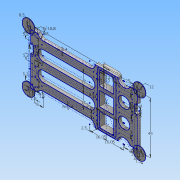
# Autodesk Inventor part: Core_top-im
Saved by Autodesk Inventor 2016 (Build 200138000, 138)
## iProperties
Created: 2015-08-27
Part Number: Core_top-im
Material: Generic
Document SubType Name: Modeling
Designer: Openlab
Density: 1 g/cm^3
Appearance: Default
Mass: 6.14664 g
Surface Area: 82.7104 cm^2
Volume: 6.14664 cm^3
Author: Openlab
Autodesk Inventor part; units mm, degrees
ref_plane "YZ Plane" through (0, 0, 0) normal (1, 0, 0) x (0, 1, 0)
ref_plane "XZ Plane" through (0, 0, 0) normal (0, 1, 0) x (-1, 0, 0)
ref_plane "XY Plane" through (0, 0, 0) normal (0, 0, 1) x (1, 0, 0)
sketch "Sketch1" plane through (0, 0, 0) normal (0, 1, 0) x (-1, 0, 0)
  line L0 (6.75, 23.75) -> (-6.75, 23.75)
  line L1 (-6.75, 23.75) -> (-6.75, 10.25)
  line L2 (-6.75, 10.25) -> (6.75, 10.25)
  line L3 (6.75, 10.25) -> (6.75, 23.75)
  line L4 (56.9183, 17) -> (21.35, 17) construction
  line L5 (69.8, -24.5) -> (69.8, -20.1) construction
  line L6 (-26.8, 24.5) -> (-26.8, -24.5) construction
  line L7 (9.25, 15.5) -> (6.75, 15.5) construction
  line L8 (6.75, 18.5) -> (9.25, 18.5) construction
  line L9 (-6.75, 15.5) -> (-9.25, 15.5) construction
  line L10 (-9.25, 18.5) -> (-6.75, 18.5) construction
  line L11 (-12.05, 18.5) -> (-24.5, 18.5) construction
  line L12 (-12.05, 15.5) -> (-24.5, 15.5) construction
  line L13 (-31, 8.5) -> (74, 8.5) construction
  line L14 (67.5, 20.5) -> (66, 20.5) construction
  line L15 (66, 13.5) -> (67.5, 13.5) construction
  line L16 (-31, 26) -> (-31, -26) construction
  line L17 (21.35, -8.5) -> (74, -8.5) construction
  line L18 (0, 20.0147) -> (0, -26) construction
  line L19 (56.8064, 0) -> (21.35, 0) construction
  line L20 (-6.75, 6.75) -> (-6.75, -6.75)
  line L21 (6.75, 6.75) -> (-6.75, 6.75)
  line L22 (6.75, -6.75) -> (6.75, 6.75)
  line L23 (-6.75, -6.75) -> (6.75, -6.75)
  line L24 (6.75, 1.5) -> (9.25, 1.5) construction
  line L25 (9.25, -1.5) -> (6.75, -1.5) construction
  line L26 (67.5, 3.5) -> (66, 3.5) construction
  line L27 (66, -3.5) -> (67.5, -3.5) construction
  line L28 (-6.75, -10.25) -> (-6.75, -23.75)
  line L29 (6.75, -10.25) -> (-6.75, -10.25)
  line L30 (6.75, -23.75) -> (6.75, -10.25)
  line L31 (-6.75, -23.75) -> (6.75, -23.75)
  line L32 (56.3008, -17) -> (21.35, -17) construction
  line L33 (67.5, -13.5) -> (66, -13.5) construction
  line L34 (66, -20.5) -> (67.5, -20.5) construction
  line L35 (9.25, -18.5) -> (6.75, -18.5) construction
  line L36 (6.75, -15.5) -> (9.25, -15.5) construction
  line L37 (74, 5) -> (72.5, 5) construction
  line L38 (69.8, 12) -> (72.5, 12) construction
  line L39 (-9.25, -15.5) -> (-6.75, -15.5) construction
  line L40 (-6.75, -18.5) -> (-9.25, -18.5) construction
  line L41 (-12.05, -18.5) -> (-24.5, -18.5) construction
  line L42 (-9.25, 1.5) -> (-6.75, 1.5) construction
  line L43 (-6.75, -1.5) -> (-9.25, -1.5) construction
  line L44 (-12.05, -1.5) -> (-24.5, -1.5) construction
  line L45 (-29.5, 5) -> (-31, 5) construction
  line L46 (-31, 12) -> (-29.5, 12) construction
  line L47 (67.5, 5.5) -> (66, 5.5) construction
  line L48 (66, 5.5) -> (66, 11.5) construction
  line L49 (66, 11.5) -> (67.5, 11.5) construction
  line L50 (-24.5, 5.5) -> (-23.5, 5.5) construction
  line L51 (-23.5, 5.5) -> (-23.5, 11.5) construction
  line L52 (-23.5, 11.5) -> (-24.5, 11.5) construction
  line L53 (-25, 24.5) -> (-25, 19) construction
  line L54 (-25, 5) -> (-25, 2) construction
  arc A0 (16.05, 13.5) -> (16.05, 3.5) centre (16.05, 8.5) ccw
  arc A1 (60, 3.5) -> (60, 13.5) centre (60, 8.5) ccw
  arc A2 (16.05, -3.5) -> (16.05, -13.5) centre (16.05, -8.5) ccw
  arc A3 (60, -13.5) -> (60, -3.5) centre (60, -8.5) ccw
  line L55 (16.05, 13.5) -> (60, 13.5)
  line L56 (16.05, 3.5) -> (60, 3.5)
  line L57 (16.05, -3.5) -> (60, -3.5)
  line L58 (16.05, -13.5) -> (60, -13.5)
  arc A4 (-16.05, -13.5) -> (-16.05, -3.5) centre (-16.05, -8.5) ccw
  line L59 (72.5, -24.5) -> (72.5, -19.6) construction
  line L60 (-29.5, 24.5) -> (-29.5, 12) construction
  arc A5 (-17, -3.5) -> (-17, -13.5) centre (-17, -8.5) ccw
  arc A6 (-17, 13.5) -> (-17, 3.5) centre (-17, 8.5) ccw
  line L61 (-16.05, -13.5) -> (-17, -13.5)
  line L62 (-17, -3.5) -> (-16.05, -3.5)
  line L63 (-17, 3.5) -> (-16.05, 3.5)
  line L64 (-16.05, 13.5) -> (-17, 13.5)
  arc A7 (-16.05, 3.5) -> (-16.05, 13.5) centre (-16.05, 8.5) ccw
  line L65 (58.8763, -15.5) -> (12.05, -15.5) construction
  line L66 (58.8763, -18.5) -> (12.05, -18.5) construction
  line L67 (58.8763, -1.5) -> (12.05, -1.5) construction
  line L68 (58.8763, 1.5) -> (12.05, 1.5) construction
  line L69 (58.8763, 15.5) -> (12.05, 15.5) construction
  line L70 (58.8763, 18.5) -> (12.05, 18.5) construction
  arc A8 (61, -14.4) -> (58.8763, -15.5) centre (61, -17) ccw construction
  arc A9 (58.8763, -18.5) -> (61, -19.6) centre (61, -17) ccw construction
  arc A10 (61, 2.6) -> (58.8763, 1.5) centre (61, 0) ccw construction
  arc A11 (58.8763, -1.5) -> (61, -2.6) centre (61, 0) ccw construction
  arc A12 (61, 19.6) -> (58.8763, 18.5) centre (61, 17) ccw construction
  arc A13 (58.8763, 15.5) -> (61, 14.4) centre (61, 17) ccw construction
  arc A14 (63.5, -26) -> (60, -22.5) centre (60, -26) ccw construction
  arc A15 (16.05, -22.5) -> (12.55, -26) centre (16.05, -26) ccw construction
  arc A16 (64.7697, -24.5) -> (60, -21) centre (60, -26) ccw construction
  line L71 (60, -21) -> (16.05, -21) construction
  line L72 (63.5, -26) -> (74, -26) construction
  line L73 (60, -22.5) -> (16.05, -22.5) construction
  arc A17 (16.05, -21) -> (11.2803, -24.5) centre (16.05, -26) ccw construction
  arc A18 (11.2803, 24.5) -> (16.05, 21) centre (16.05, 26) ccw construction
  arc A19 (12.55, 26) -> (16.05, 22.5) centre (16.05, 26) ccw construction
  line L74 (60, 22.5) -> (16.05, 22.5) construction
  line L75 (60, 21) -> (16.05, 21) construction
  line L76 (64.7697, 24.5) -> (69.8, 24.5) construction
  line L77 (74, 26) -> (63.5, 26) construction
  arc A20 (60, 22.5) -> (63.5, 26) centre (60, 26) ccw construction
  arc A21 (60, 21) -> (64.7697, 24.5) centre (60, 26) ccw construction
  arc A22 (-12.55, -26) -> (-16.05, -22.5) centre (-16.05, -26) ccw construction
  arc A23 (-17, -22.5) -> (-20.5, -26) centre (-17, -26) ccw construction
  line L78 (-16.05, -21) -> (-17, -21) construction
  line L79 (-16.05, -22.5) -> (-17, -22.5) construction
  arc A24 (-17, -21) -> (-21.7697, -24.5) centre (-17, -26) ccw construction
  arc A25 (-11.2803, -24.5) -> (-16.05, -21) centre (-16.05, -26) ccw construction
  line L80 (11.2803, -24.5) -> (-11.2803, -24.5) construction
  line L81 (-21.7697, -24.5) -> (-29.5, -24.5) construction
  line L82 (-31, -26) -> (-20.5, -26) construction
  line L83 (-12.55, -26) -> (12.55, -26) construction
  line L84 (-16.05, 21) -> (-17, 21) construction
  line L85 (-16.05, 22.5) -> (-17, 22.5) construction
  arc A26 (-20.5, 26) -> (-17, 22.5) centre (-17, 26) ccw construction
  arc A27 (-16.05, 22.5) -> (-12.55, 26) centre (-16.05, 26) ccw construction
  arc A28 (-21.7697, 24.5) -> (-17, 21) centre (-17, 26) ccw construction
  arc A29 (-16.05, 21) -> (-11.2803, 24.5) centre (-16.05, 26) ccw construction
  line L86 (12.55, 26) -> (-12.55, 26) construction
  line L87 (-20.5, 26) -> (-31, 26) construction
  line L88 (-29.5, 24.5) -> (-21.7697, 24.5) construction
  line L89 (-11.2803, 24.5) -> (11.2803, 24.5) construction
  line L90 (11.2803, -24.5) -> (11.2803, -26) construction
  line L91 (-11.2803, -24.5) -> (-11.2803, -26) construction
  line L92 (-11.2803, 24.5) -> (-11.2803, 26) construction
  line L93 (11.2803, 24.5) -> (11.2803, 26) construction
  line L94 (72.5, 12) -> (74, 12) construction
  line L95 (72.5, 5) -> (69.8, 5) construction
  line L96 (-26.8, 12) -> (-29.5, 12) construction
  line L97 (-26.8, 5) -> (-29.5, 5) construction
  line L98 (11.55, -21) -> (9.75, -21) construction
  line L99 (9.75, -13) -> (11.55, -13) construction
  line L100 (11.55, -4) -> (9.75, -4) construction
  line L101 (9.75, 4) -> (11.55, 4) construction
  line L102 (11.55, 13) -> (9.75, 13) construction
  line L103 (9.75, 21) -> (11.55, 21) construction
  line L104 (-9.75, -21) -> (-11.55, -21) construction
  line L105 (-11.55, -13) -> (-9.75, -13) construction
  line L106 (-9.75, -4) -> (-11.55, -4) construction
  line L107 (-11.55, 4) -> (-9.75, 4) construction
  line L108 (-9.75, 13) -> (-11.55, 13) construction
  line L109 (-11.55, 21) -> (-9.75, 21) construction
  line L110 (11.55, -13) -> (11.55, -15) construction
  line L111 (11.55, -19) -> (11.55, -21) construction
  line L112 (9.75, -21) -> (9.75, -19) construction
  line L113 (9.75, -15) -> (9.75, -13) construction
  line L114 (11.55, 4) -> (11.55, 2) construction
  line L115 (11.55, -2) -> (11.55, -4) construction
  line L116 (9.75, -4) -> (9.75, -2) construction
  line L117 (9.75, 2) -> (9.75, 4) construction
  line L118 (11.55, 21) -> (11.55, 19) construction
  line L119 (11.55, 15) -> (11.55, 13) construction
  line L120 (9.75, 13) -> (9.75, 15) construction
  line L121 (9.75, 19) -> (9.75, 21) construction
  line L122 (-9.75, -13) -> (-9.75, -15) construction
  line L123 (-9.75, -19) -> (-9.75, -21) construction
  line L124 (-11.55, -21) -> (-11.55, -19) construction
  line L125 (-11.55, -15) -> (-11.55, -13) construction
  line L126 (-9.75, 4) -> (-9.75, 2) construction
  line L127 (-9.75, -2) -> (-9.75, -4) construction
  line L128 (-11.55, -4) -> (-11.55, -2) construction
  line L129 (-11.55, 2) -> (-11.55, 4) construction
  line L130 (-9.75, 21) -> (-9.75, 19) construction
  line L131 (-9.75, 15) -> (-9.75, 13) construction
  line L132 (-11.55, 13) -> (-11.55, 15) construction
  line L133 (-11.55, 19) -> (-11.55, 21) construction
  line L134 (67.5, -11.5) -> (66, -11.5) construction
  line L135 (66, -11.5) -> (66, -5.5) construction
  line L136 (66, -5.5) -> (67.5, -5.5) construction
  line L137 (68, -21) -> (68, -24.5) construction
  arc A30 (9.75, -19) -> (9.25, -18.5) centre (9.25, -19) ccw construction
  arc A31 (12.05, -18.5) -> (11.55, -19) centre (12.05, -19) ccw construction
  arc A32 (11.55, -15) -> (12.05, -15.5) centre (12.05, -15) ccw construction
  arc A33 (9.25, -15.5) -> (9.75, -15) centre (9.25, -15) ccw construction
  arc A34 (9.75, -2) -> (9.25, -1.5) centre (9.25, -2) ccw construction
  arc A35 (12.05, -1.5) -> (11.55, -2) centre (12.05, -2) ccw construction
  arc A36 (11.55, 2) -> (12.05, 1.5) centre (12.05, 2) ccw construction
  arc A37 (9.25, 1.5) -> (9.75, 2) centre (9.25, 2) ccw construction
  arc A38 (9.75, 15) -> (9.25, 15.5) centre (9.25, 15) ccw construction
  arc A39 (12.05, 15.5) -> (11.55, 15) centre (12.05, 15) ccw construction
  arc A40 (11.55, 19) -> (12.05, 18.5) centre (12.05, 19) ccw construction
  arc A41 (9.25, 18.5) -> (9.75, 19) centre (9.25, 19) ccw construction
  arc A42 (-9.75, 19) -> (-9.25, 18.5) centre (-9.25, 19) ccw construction
  arc A43 (-12.05, 18.5) -> (-11.55, 19) centre (-12.05, 19) ccw construction
  arc A44 (-11.55, 15) -> (-12.05, 15.5) centre (-12.05, 15) ccw construction
  arc A45 (-9.25, 15.5) -> (-9.75, 15) centre (-9.25, 15) ccw construction
  arc A46 (-9.75, 2) -> (-9.25, 1.5) centre (-9.25, 2) ccw construction
  arc A47 (-12.05, 1.5) -> (-11.55, 2) centre (-12.05, 2) ccw construction
  arc A48 (-11.55, -2) -> (-12.05, -1.5) centre (-12.05, -2) ccw construction
  arc A49 (-9.25, -1.5) -> (-9.75, -2) centre (-9.25, -2) ccw construction
  arc A50 (-9.75, -15) -> (-9.25, -15.5) centre (-9.25, -15) ccw construction
  arc A51 (-12.05, -15.5) -> (-11.55, -15) centre (-12.05, -15) ccw construction
  arc A52 (-9.25, -18.5) -> (-9.75, -19) centre (-9.25, -19) ccw construction
  arc A53 (-11.55, -19) -> (-12.05, -18.5) centre (-12.05, -19) ccw construction
  line L138 (65.5, -19.6) -> (61, -19.6) construction
  line L139 (66, -13.5) -> (66, -13.9) construction
  line L140 (61, -14.4) -> (65.5, -14.4) construction
  line L141 (65.5, -2.6) -> (61, -2.6) construction
  line L142 (66, 3.5) -> (66, 3.1) construction
  line L143 (66, -3.1) -> (66, -3.5) construction
  line L144 (61, 2.6) -> (65.5, 2.6) construction
  line L145 (65.5, 14.4) -> (61, 14.4) construction
  line L146 (66, 20.5) -> (66, 20.1) construction
  line L147 (66, 13.9) -> (66, 13.5) construction
  line L148 (61, 19.6) -> (65.5, 19.6) construction
  arc A54 (65.5, -14.4) -> (66, -13.9) centre (65.5, -13.9) ccw construction
  arc A55 (68, -12) -> (67.5, -11.5) centre (67.5, -12) ccw construction
  arc A56 (67.5, -5.5) -> (68, -5) centre (67.5, -5) ccw construction
  arc A57 (68, 5) -> (67.5, 5.5) centre (67.5, 5) ccw construction
  arc A58 (67.5, 11.5) -> (68, 12) centre (67.5, 12) ccw construction
  arc A59 (66, -3.1) -> (65.5, -2.6) centre (65.5, -3.1) ccw construction
  arc A60 (65.5, 2.6) -> (66, 3.1) centre (65.5, 3.1) ccw construction
  arc A61 (66, 13.9) -> (65.5, 14.4) centre (65.5, 13.9) ccw construction
  arc A62 (65.5, 19.6) -> (66, 20.1) centre (65.5, 20.1) ccw construction
  line L149 (72.5, -2.6) -> (72.5, 2.6) construction
  line L150 (72.5, -2.6) -> (70.3, -2.6) construction
  line L151 (66, -20.5) -> (66, -20.1) construction
  arc A63 (66, -20.1) -> (65.5, -19.6) centre (65.5, -20.1) ccw construction
  line L152 (68, -13) -> (68, -12) construction
  line L153 (68, 4) -> (68, 5) construction
  line L154 (68, 21) -> (68, 24.5) construction
  line L155 (72.5, -19.6) -> (72.5, -14.4) construction
  line L156 (72.5, -19.6) -> (70.3, -19.6) construction
  line L157 (72.5, -24.5) -> (69.8, -24.5) construction
  line L158 (69.8, -24.5) -> (68, -24.5) construction
  line L159 (68, -24.5) -> (64.7697, -24.5) construction
  line L160 (70.3, -14.4) -> (72.5, -14.4) construction
  line L161 (72.5, -14.4) -> (72.5, -2.6) construction
  line L162 (69.8, -13.9) -> (69.8, -3.1) construction
  line L163 (68, -4) -> (68, -5) construction
  line L164 (72.5, 2.6) -> (72.5, 5) construction
  line L165 (70.3, 2.6) -> (72.5, 2.6) construction
  line L166 (69.8, 3.1) -> (69.8, 5) construction
  line L167 (72.5, 14.4) -> (72.5, 19.6) construction
  line L168 (72.5, 14.4) -> (70.3, 14.4) construction
  line L169 (74, -26) -> (74, 26) construction
  line L170 (72.5, 19.6) -> (72.5, 24.5) construction
  line L171 (69.8, 20.1) -> (69.8, 24.5) construction
  line L172 (70.3, 19.6) -> (72.5, 19.6) construction
  line L173 (72.5, 12) -> (72.5, 14.4) construction
  line L174 (69.8, 24.5) -> (72.5, 24.5) construction
  line L175 (69.8, 12) -> (69.8, 13.9) construction
  line L176 (68, 13) -> (68, 12) construction
  arc A64 (67.5, -13.5) -> (68, -13) centre (67.5, -13) ccw construction
  arc A65 (68, -4) -> (67.5, -3.5) centre (67.5, -4) ccw construction
  arc A66 (67.5, 3.5) -> (68, 4) centre (67.5, 4) ccw construction
  arc A67 (68, 13) -> (67.5, 13.5) centre (67.5, 13) ccw construction
  arc A68 (67.5, 20.5) -> (68, 21) centre (67.5, 21) ccw construction
  arc A69 (70.3, -19.6) -> (69.8, -20.1) centre (70.3, -20.1) ccw construction
  arc A70 (69.8, -13.9) -> (70.3, -14.4) centre (70.3, -13.9) ccw construction
  arc A71 (70.3, -2.6) -> (69.8, -3.1) centre (70.3, -3.1) ccw construction
  arc A72 (69.8, 3.1) -> (70.3, 2.6) centre (70.3, 3.1) ccw construction
  arc A73 (70.3, 14.4) -> (69.8, 13.9) centre (70.3, 13.9) ccw construction
  arc A74 (69.8, 20.1) -> (70.3, 19.6) centre (70.3, 20.1) ccw construction
  line L177 (69.8, 5) -> (69.8, 12) construction
  line L178 (-25, 15) -> (-25, 12) construction
  line L179 (-24.5, 1.5) -> (-12.05, 1.5) construction
  line L180 (-25, -2) -> (-25, -15) construction
  line L181 (-25, -19) -> (-25, -24.5) construction
  line L182 (-24.5, -15.5) -> (-12.05, -15.5) construction
  line L183 (-29.5, 5) -> (-29.5, -24.5) construction
  arc A75 (-25, 19) -> (-24.5, 18.5) centre (-24.5, 19) ccw construction
  arc A76 (-24.5, 15.5) -> (-25, 15) centre (-24.5, 15) ccw construction
  arc A77 (-25, 12) -> (-24.5, 11.5) centre (-24.5, 12) ccw construction
  arc A78 (-24.5, 5.5) -> (-25, 5) centre (-24.5, 5) ccw construction
  arc A79 (-25, 2) -> (-24.5, 1.5) centre (-24.5, 2) ccw construction
  arc A80 (-24.5, -1.5) -> (-25, -2) centre (-24.5, -2) ccw construction
  arc A81 (-25, -15) -> (-24.5, -15.5) centre (-24.5, -15) ccw construction
  arc A82 (-24.5, -18.5) -> (-25, -19) centre (-24.5, -19) ccw construction
  arc A83 (68, -21) -> (67.5, -20.5) centre (67.5, -21) ccw construction
  line L184 (-29.1, 23.6) -> (-29.1, 12.9)
  line L185 (-28.6, 12.4) -> (-26.4, 12.4)
  line L186 (-26.4, 12.4) -> (-26.4, 4.6)
  line L187 (-26.4, 4.6) -> (-28.6, 4.6)
  line L188 (-29.1, 4.1) -> (-29.1, -23.6)
  line L189 (-28.6, -24.1) -> (-22.3898, -24.1)
  line L190 (-10.9953, 24.1) -> (10.9953, 24.1) construction
  line L191 (16.05, 20.6) -> (60, 20.6)
  line L192 (65.3898, 24.1) -> (71.6, 24.1)
  line L193 (72.1, 23.6) -> (72.1, 12.9)
  line L194 (71.6, 12.4) -> (69.4, 12.4)
  line L195 (69.4, 12.4) -> (69.4, 4.6)
  line L196 (69.4, 4.6) -> (71.6, 4.6)
  line L197 (72.1, 4.1) -> (72.1, -23.6)
  line L198 (71.6, -24.1) -> (65.3898, -24.1)
  line L199 (60.0007, -20.6) -> (16.05, -20.6)
  line L200 (-10.9953, -24.1) -> (10.9953, -24.1) construction
  arc A84 (10.9953, 24.1) -> (16.05, 20.6) centre (16.05, 26) ccw
  arc A85 (16.05, -20.6) -> (10.9953, -24.1) centre (16.05, -26) ccw
  arc A86 (-16.05, 20.6) -> (-10.9953, 24.1) centre (-16.05, 26) ccw
  arc A87 (-21.933, 23.8034) -> (-17, 20.6) centre (-17, 26) ccw
  arc A88 (-10.9953, -24.1) -> (-16.05, -20.6) centre (-16.05, -26) ccw
  arc A89 (60, 20.6) -> (64.933, 23.8034) centre (60, 26) ccw
  arc A90 (64.933, -23.8034) -> (60, -20.6) centre (60, -26) ccw
  line L201 (-22.3898, 24.1) -> (-28.6, 24.1)
  line L202 (-17, 20.6) -> (-16.05, 20.6)
  arc A91 (-17, -20.6) -> (-21.933, -23.8034) centre (-17, -26) ccw
  line L203 (-17, -20.6) -> (-16.05, -20.6)
  line L204 (-10.9953, 24.1) -> (-10.9953, 25.5)
  line L205 (10.9953, 24.1) -> (10.9953, 25.5)
  line L206 (10.4953, 26) -> (-10.4953, 26)
  line L207 (10.9953, -24.1) -> (10.9953, -25.5)
  line L208 (-10.9953, -24.1) -> (-10.9953, -25.5)
  line L209 (10.4953, -26) -> (-10.4953, -26)
  arc A92 (72.1, 23.6) -> (71.6, 24.1) centre (71.6, 23.6) ccw
  arc A93 (71.6, 12.4) -> (72.1, 12.9) centre (71.6, 12.9) ccw
  arc A94 (72.1, 4.1) -> (71.6, 4.6) centre (71.6, 4.1) ccw
  arc A95 (71.6, -24.1) -> (72.1, -23.6) centre (71.6, -23.6) ccw
  arc A96 (10.4953, -26) -> (10.9953, -25.5) centre (10.4953, -25.5) ccw
  arc A97 (-10.9953, -25.5) -> (-10.4953, -26) centre (-10.4953, -25.5) ccw
  arc A98 (-29.1, -23.6) -> (-28.6, -24.1) centre (-28.6, -23.6) ccw
  arc A99 (-28.6, 4.6) -> (-29.1, 4.1) centre (-28.6, 4.1) ccw
  arc A100 (-29.1, 12.9) -> (-28.6, 12.4) centre (-28.6, 12.9) ccw
  arc A101 (-28.6, 24.1) -> (-29.1, 23.6) centre (-28.6, 23.6) ccw
  arc A102 (-10.4953, 26) -> (-10.9953, 25.5) centre (-10.4953, 25.5) ccw
  arc A103 (10.9953, 25.5) -> (10.4953, 26) centre (10.4953, 25.5) ccw
  arc A104 (64.933, -23.8034) -> (65.3898, -24.1) centre (65.3898, -23.6) ccw
  arc A105 (-22.3898, -24.1) -> (-21.933, -23.8034) centre (-22.3898, -23.6) ccw
  arc A106 (-21.933, 23.8034) -> (-22.3898, 24.1) centre (-22.3898, 23.6) ccw
  arc A107 (65.3898, 24.1) -> (64.933, 23.8034) centre (65.3898, 23.6) ccw
  line L210 (-6.25, -25.75) -> (6.25, -25.75)
  line L211 (8.75, -23.25) -> (8.75, 23.25)
  line L212 (6.25, 25.75) -> (-6.25, 25.75)
  line L213 (-8.75, 23.25) -> (-8.75, -23.25)
  line L214 (-8.75, -25.75) -> (8.75, 25.75) construction
  line L215 (8.75, -25.75) -> (-8.75, 25.75) construction
  arc A108 (6.25, -25.75) -> (8.75, -23.25) centre (6.25, -23.25) ccw
  arc A109 (8.75, 23.25) -> (6.25, 25.75) centre (6.25, 23.25) ccw
  arc A110 (-6.25, 25.75) -> (-8.75, 23.25) centre (-6.25, 23.25) ccw
  arc A111 (-8.75, -23.25) -> (-6.25, -25.75) centre (-6.25, -23.25) ccw
  circle A112 centre (-31, -26) radius 6
  circle A113 centre (-31, 26) radius 6
  circle A114 centre (74, -26) radius 6
  circle A115 centre (74, 26) radius 6
  point P0 (0, 0)
  point P1 (0, -17)
  point P2 (0, 0)
  point P3 (0, 17)
  point P4 (72.5, -8.5)
  dimension "d0" = 7
  dimension "d4" = 6
  dimension "d5" = 6
  dimension "d6" = 5
  dimension "d7" = 1.5
  dimension "d8" = 1.5
  dimension "d9" = 1.5
  dimension "d12" = 2.7
  dimension "d13" = 2.7
  dimension "d14" = 7
  dimension "d15" = 7
  dimension "d16" = 25
  dimension "d17" = 5
  dimension "d18" = 1.8
  dimension "d19" = 8
  dimension "d20" = 3
  dimension "d23" = 13.5
  dimension "d26" = 8
  dimension "d27" = 7
  dimension "d28" = 7
  dimension "d29" = 2
  dimension "d30" = 1.8
  dimension "d31" = 8
  dimension "d32" = 1.8
  dimension "d33" = 2.7
  dimension "d34" = 1.5
  dimension "d35" = 3
  dimension "d36" = 3
  dimension "d37" = 3
  dimension "d38" = 3
  dimension "d39" = 0.5
  dimension "d40" = 68
  dimension "d41" = 5.2
  dimension "d42" = 7
  dimension "d43" = 5.2
  dimension "d44" = 5.2
  dimension "d45" = 1.5
  dimension "d46" = 1.5
  dimension "sb" = 0.4
  dimension "d48" = 0.4
  dimension "d49" = 0.4
  dimension "d50" = 0.4
  dimension "d51" = 0.4
  dimension "d52" = 0.4
  dimension "d54" = 0.4
  dimension "d55" = 0.4
  dimension "d56" = 0.4
  dimension "d57" = 0.4
  dimension "d58" = 10.8
  dimension "d71" = 0.5
  dimension "d76" = 2
  dimension "d77" = 2
  dimension "d78" = 2.5
  dimension "d81" = 17
  dimension "d82" = 17
  dimension "d83" = 49
  dimension "d87" = 12
  dimension "d88" = 16.05
  dimension "d89" = 16.05
  dimension "d90" = 13.5
  constraints: 434 end point, 226 point on circle, 187 tangent, 158 perpendicular, 116 centre point, 103 equal radius, 93 collinear, 62 point on line, 55 parallel, 32 horizontal, 22 coincident, 14 vertical alignment, 7 horizontal alignment, 4 midpoint, 2 vertical, 38 other
  measures "d0" distance of L14.end L15.start
  measures "d4" distance of L47.end L48.end
  measures "d5" distance of L50.end L51.end
  measures "d6" radius of A16
  measures "d7" radial gap between concentric circles of A14 A16
  measures "d8" distance between parallel lines of L77 L76
  measures "d9" distance between parallel lines of L81 L82
  measures "d12" distance between parallel lines of L60 L6
  measures "d13" distance between parallel lines of L5 L59
  measures "d14" distance between parallel lines of L95 L38
  measures "d15" distance between parallel lines of L97 L96
  measures "d16" distance between parallel lines of L53 L18
  measures "d17" radius of A2
  measures "d18" distance of L98.start L98.end
  measures "d19" distance between parallel lines of L99 L98
  measures "d20" distance between parallel lines of L30 L113
  measures "d23" distance between parallel lines of L1 L3
  measures "d26" distance from line of A14.centre L137
  measures "d27" distance between parallel lines of L26 L27
  measures "d28" distance between parallel lines of L33 L34
  measures "d29" distance between parallel lines of L48 L153
  measures "d30" distance between parallel lines of L137 L5
  measures "d31" distance from line of L181 A24.centre
  measures "d32" distance between parallel lines of L6 L181
  measures "d33" distance between parallel lines of L183 L6
  measures "d34" distance between parallel lines of L16 L183
  measures "d35" distance between parallel lines of L182 L41
  measures "d36" distance between parallel lines of L44 L179
  measures "d37" distance between parallel lines of L11 L12
  measures "d38" distance between parallel lines of L122 L28
  measures "d39" radius of A34
  measures "d40" distance between parallel lines of L154 L18
  measures "d41" distance between parallel lines of L160 L156
  measures "d42" distance from line of A10.centre L163
  measures "d43" distance between parallel lines of L165 L150
  measures "d44" distance between parallel lines of L172 L168
  measures "d45" distance between parallel lines of L54 L51
  measures "d46" distance between parallel lines of L59 L169
  measures "sb" distance between parallel lines of L60 L184
  measures "d48" distance between parallel lines of L88 L201
  measures "d49" distance between parallel lines of L96 L185
  measures "d50" distance between parallel lines of L6 L186
  measures "d51" distance between parallel lines of L187 L97
  measures "d52" distance between parallel lines of L81 L189
  measures "d54" distance between parallel lines of L75 L191
  measures "d55" distance between parallel lines of L71 L199
  measures "d56" distance between parallel lines of L170 L193
  measures "d57" distance between parallel lines of L195 L177
  measures "d58" diameter of A89
  measures "d71" radius of A92
  measures "d76" distance between parallel lines of L212 L0
  measures "d77" distance between parallel lines of L213 L1
  measures "d78" radius of A108
  measures "d81" distance between parallel lines of L19 L4
  measures "d82" distance between parallel lines of L32 L19
  measures "d83" distance between parallel lines of L81 L88
  measures "d87" diameter of A113
  measures "d88" distance from line of L18 A17.centre
  measures "d89" distance from line of L18 A25.centre
  measures "d90" distance between parallel lines of L2 L0
extrude "Extrusion1" add sketch "Sketch1" along normal blind 3 contours A101 L201 A113 L184 | A113 L201 A106 A87 L202 A86 L204 A102 L206 A103 L205 A84 L191 A89 A107 L192 A115 L193 A93 L194 L195 L196 A94 L197 A114 L198 A104 A90 L199 A85 L207 A96 L209 A97 L208 A88 L203 A91 A105 L189 A112 L188 A99 L187 L186 L185 A100 L184 | A112 L189 A98 L188 | L192 A92 L193 A115 | A114 L197 A95 L198 | A111 L213 A110 L212 A109 L211 A108 L210 picked at (-26.6019, 23.6815) picked at (-26.6019, -23.6815) picked at (71.6815, 21.6019) picked at (71.6815, -21.6019)
sketch "Sketch2" plane through (0, 3, 0) normal (0, 1, 0) x (1, 0, 0)
  arc A0 (-60, 13.5) -> (-60, 3.5) centre (-60, 8.5) ccw projected
  line L0 (-60, 13.5) -> (-16.05, 13.5) projected
  arc A1 (-16.05, 3.5) -> (-16.05, 13.5) centre (-16.05, 8.5) ccw projected
  line L1 (-16.05, 3.5) -> (-60, 3.5) projected
  line L2 (-60, -3.5) -> (-16.05, -3.5) projected
  arc A2 (-60, -3.5) -> (-60, -13.5) centre (-60, -8.5) ccw projected
  line L3 (-16.05, -13.5) -> (-60, -13.5) projected
  arc A3 (-16.05, -13.5) -> (-16.05, -3.5) centre (-16.05, -8.5) ccw projected
  arc A4 (16.05, 13.5) -> (16.05, 3.5) centre (16.05, 8.5) ccw projected
  line L4 (16.05, 13.5) -> (17, 13.5) projected
  arc A5 (17, 3.5) -> (17, 13.5) centre (17, 8.5) ccw projected
  line L5 (17, 3.5) -> (16.05, 3.5) projected
  arc A6 (16.05, -3.5) -> (16.05, -13.5) centre (16.05, -8.5) ccw projected
  line L6 (16.05, -3.5) -> (17, -3.5) projected
  arc A7 (17, -13.5) -> (17, -3.5) centre (17, -8.5) ccw projected
  line L7 (17, -13.5) -> (16.05, -13.5) projected
  arc A8 (-60, 12.5) -> (-60, 4.5) centre (-60, 8.5) ccw
  arc A9 (-16.05, 4.5) -> (-16.05, 12.5) centre (-16.05, 8.5) ccw
  arc A10 (-60, -4.5) -> (-60, -12.5) centre (-60, -8.5) ccw
  arc A11 (-16.05, -12.5) -> (-16.05, -4.5) centre (-16.05, -8.5) ccw
  arc A12 (16.05, 12.5) -> (16.525, 4.5283) centre (16.05, 8.5) ccw
  arc A13 (16.525, 4.5283) -> (17, 12.5) centre (17, 8.5) ccw
  arc A14 (16.05, -4.5) -> (16.05, -12.5) centre (16.05, -8.5) ccw
  arc A15 (17, -12.5) -> (17, -4.5) centre (17, -8.5) ccw
  line L8 (16.05, -4.5) -> (17, -4.5)
  line L9 (16.05, -12.5) -> (17, -12.5)
  line L10 (16.05, 12.5) -> (17, 12.5)
  line L11 (-60, 12.5) -> (-16.05, 12.5)
  line L12 (-60, 4.5) -> (-16.05, 4.5)
  line L13 (-60, -4.5) -> (-16.05, -4.5)
  line L14 (-60, -12.5) -> (-16.05, -12.5)
  point P0 (0, 0)
  dimension "d63" = 8
  constraints: 16 point on circle, 14 end point, 9 tangent, 8 centre point, 8 coincident, 7 equal radius, 3 parallel, 2 horizontal
  measures "d63" diameter of A9
extrude "Extrusion2" [suppressed]
extrude "Extrusion3" add sketch "Sketch1" along normal blind 5.5 contours A111 L213 A110 L212 A109 L211 A108 L210
extrude "Extrusion4" add sketch "Sketch1" along normal blind 0.5 contours A101 L201 A113 L184 | L184 A113 L201 A101 | A112 L189 A98 L188 | L188 A98 L189 A112 | A115 L193 A92 L192 | L192 A92 L193 A115 | A114 L197 A95 L198 | L198 A95 L197 A114
equation "\"d48\" = sb"
equation "\"d49\" = sb"
equation "\"d50\" = sb"
equation "\"d51\" = sb"
equation "\"d52\" = sb"
equation "\"d54\" = sb"
equation "\"d55\" = sb"
equation "\"d56\" = sb"
equation "\"d57\" = sb"
body "Solid1"
